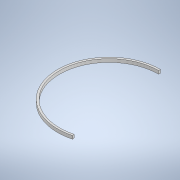
# Autodesk Inventor part: przestrzeń robocza
Saved by Autodesk Inventor 2022 (Build 260153000, 153)
## iProperties
Created: 2022-06-13
Part Number: przestrzeń robocza
Material: Ogólny
Document SubType Name: Sheet Metal
Designer: admin
Density: 1 g/cm^3
Sheet Metal Rule: Domyślny_mm
Appearance: Domyślna
Author: admin
Autodesk Inventor part; units mm, degrees
ref_plane "YZ Plane" through (0, 0, 0) normal (1, 0, 0) x (0, 1, 0)
ref_plane "XZ Plane" through (0, 0, 0) normal (0, 1, 0) x (-1, 0, 0)
ref_plane "XY Plane" through (0, 0, 0) normal (0, 0, 1) x (1, 0, 0)
sketch "Szkic1" plane through (0, 0, 0) normal (0, 1, 0) x (-1, 0, 0)
  arc A0 (0, -1101.314) -> (-285.041, 1063.7876) centre (0, 0) ccw
  line L0 (0, -1060) -> (0, -1101.314)
  line L1 (-274.3482, 1023.8814) -> (-285.041, 1063.7876)
  arc A1 (0, -1060) -> (-274.3482, 1023.8814) centre (0, 0) ccw
  line L2 (0, 0) -> (-274.3482, 1023.8814)
  dimension "d0" = 2202.628
  dimension "d1" = 195
  dimension "d2" = 2120
  dimension "d5" = 41.314
  constraints: 6 end point, 4 point on circle, 2 centre point, 2 coincident, 1 collinear, 1 vertical
  measures "d0" diameter of A0
  measures "d2" diameter of A1
  measures "d5" distance of L0.start L0.end
extrude "Wyciągnięcie proste1" add sketch "Szkic1" along normal blind 68.225
equation "\"PromieńGięcia\" = Grubość"
equation "\"SzerokośćGięciaPodcięcia\" = Grubość"
equation "\"GłębokośćGięciaPodcięcia\" = 0.5 * Grubość"
equation "\"RozmiarPodcięciaNarożnika\" = 4 * Grubość"
equation "\"MinimalnaPozostałość\" = 2 * Grubość"
equation "\"PromieńPrzejścia\" = PromieńGięcia"
equation "\"Rozmiar_promienia_Jacobiego\" = PromieńGięcia"
equation "\"Wielk_odstępu\" = Grubość"
equation "\"Grubość\" = 0.5"
